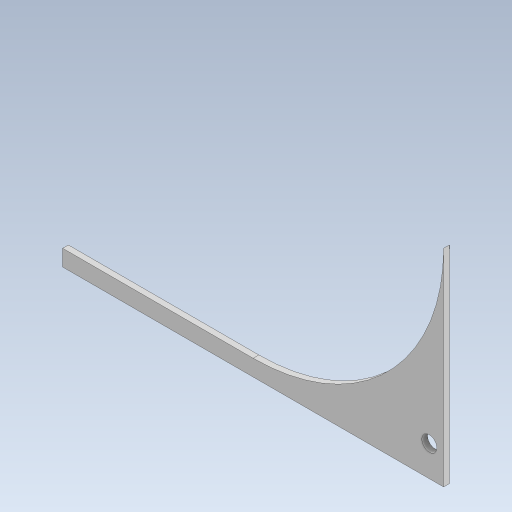
# Autodesk Inventor part: 零件9
Saved by Autodesk Inventor 2023 (Build 270158000, 158)
## iProperties
Created: 2023-05-16
Part Number: 零件9
Material: 一般
Document SubType Name: Modeling
Designer: Johnny Jou
Density: 1 g/cm^3
Appearance: 預設
Author: Johnny Jou
Autodesk Inventor part; units mm, degrees
ref_plane "YZ Plane" through (0, 0, 0) normal (1, 0, 0) x (0, 1, 0)
ref_plane "XZ Plane" through (0, 0, 0) normal (0, 1, 0) x (-1, 0, 0)
ref_plane "XY Plane" through (0, 0, 0) normal (0, 0, 1) x (1, 0, 0)
sketch "草圖1" plane through (0, 0, 0) normal (0, 0, 1) x (1, 0, 0)
  line L0 (0, -80) -> (100, -80)
  arc A0 (100, -80) -> (200, 20) centre (100, 20) ccw
  line L1 (200, 20) -> (200, 40)
  line L2 (200, 40) -> (100, 40)
  line L3 (100, 40) -> (100, -80)
  line L4 (100, -80) -> (200, -80)
  line L5 (200, -80) -> (200, 40)
  line L6 (215, -80) -> (200, -80)
  circle A1 centre (192.5, -72.5) radius 7.5
  circle A2 centre (192.5, -72.5) radius 4
  line L7 (200, -80) -> (0, -80)
  line L8 (0, -80) -> (0, -88.525)
  line L9 (0, -88.525) -> (200, -88.525)
  line L10 (200, -88.525) -> (200, -80)
  point P0 (200, 20)
  point P1 (200, -72.5)
  point P2 (192.5, -80)
  dimension "d4" = 15
  dimension "d5" = 8
  dimension "d6" = 8.525
  constraints: 22 end point, 4 parallel, 3 centre point, 3 horizontal, 2 coincident, 2 collinear, 2 perpendicular, 2 point on circle, 2 tangent, 1 vertical, 1 vertical alignment, 5 other
  measures "d4" diameter of A1
  measures "d5" diameter of A2
  measures "d6" distance between parallel lines of L4 L9
extrude "擠出1" add sketch "草圖1" along normal blind 3 contours L0 L4 L10 L9 L8 | A0 L5 A1 L4 | A1 L5 L4 | A1
